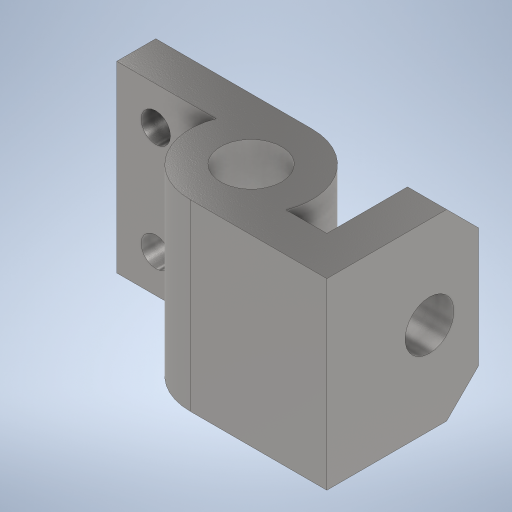
# Autodesk Inventor part: practice4
Saved by Autodesk Inventor 2024 (Build 280153000, 153)
## iProperties
Created: 2024-02-15
Part Number: practice4
Material: Stahl, galvanisiert
Document SubType Name: Modeling
Designer: ffogue
Density: 7.85 g/cm^3
Appearance: Galvanisiert
Author: ffogue
Autodesk Inventor part; units mm, degrees
ref_plane "YZ Plane" through (0, 0, 0) normal (1, 0, 0) x (0, 1, 0)
ref_plane "XZ Plane" through (0, 0, 0) normal (0, 1, 0) x (-1, 0, 0)
ref_plane "XY Plane" through (0, 0, 0) normal (0, 0, 1) x (1, 0, 0)
sketch "Skizze1" plane through (0, 0, 0) normal (0, 0, 1) x (1, 0, 0)
  line L0 (40, 37) -> (56, 37)
  line L1 (56, 37) -> (56, -25)
  line L2 (40, -9) -> (40, 37)
  line L3 (56, -25) -> (0, -25)
  line L4 (40, -9) -> (23.3238, -9)
  line L5 (0, 25) -> (-64, 25)
  line L6 (-64, 25) -> (-64, 9)
  line L7 (-64, 9) -> (-23.3238, 9)
  arc A0 (23.3238, -9) -> (0, 25) centre (0, 0) ccw
  arc A1 (-23.3238, 9) -> (0, -25) centre (0, 0) ccw
  dimension "d0" = 16
  dimension "d1" = 25
  dimension "d2" = 62
  dimension "d3" = 56
  dimension "d4" = 16
  dimension "d5" = 120
  dimension "d6" = 16
  dimension "d7" = 25
  constraints: 16 end point, 4 horizontal, 4 point on circle, 3 perpendicular, 2 centre point, 2 tangent, 1 coincident, 1 parallel
  measures "d0" distance between parallel lines of L3 L4
  measures "d1" distance from line of L3 A0.centre
  measures "d2" distance between parallel lines of L0 L3
  measures "d3" distance from line of L1 A0.centre
  measures "d4" distance between parallel lines of L1 L2
  measures "d5" distance between parallel lines of L1 L6
  measures "d6" distance between parallel lines of L7 L5
  measures "d7" radius of A0
extrude "Extrusion1" add sketch "Skizze1" along normal blind 75
sketch "Skizze2" plane through (0, 0, 75) normal (0, 0, 1) x (1, 0, 0)
  circle A0 centre (0, 0) radius 12.5
  dimension "d10" = 25
  constraints: 1 centre point, 1 coincident
  measures "d10" diameter of A0
extrude "Extrusion2" cut sketch "Skizze2" against normal up to surface (75 mm away)
chamfer "Fasen1" distance 13 angle 45 2 edges at (48, 37, 75) (48, 37, 0)
sketch "Skizze3" plane through (56, -25, 75) normal (1, 0, 0) x (0, 0, -1)
  line L0 (62, 62) -> (13, 62) projected
  point P0 (75, 25)
  point P1 (37.5, 42)
  point P2 (37.5, 62)
  dimension "d23" = 20
  constraints: 1 midpoint, 1 vertical alignment
  measures "d23" distance from line of point (37.5, 42) L0
hole "Bohrung1" at (56, 17, 37.5) direction (-1, 0, 0) diameter 20 depth 16
sketch "Skizze4" plane through (-64, 25, 0) normal (0, 1, 0) x (1, 0, 0)
  line L0 (0, 0) -> (0, -75) projected
  line L1 (0, -37.5) -> (64, -37.5) construction
  line L2 (64, 0) -> (64, -75) projected
  point P0 (16, -59.5)
  point P1 (16, -15.5)
  dimension "d31" = 44
  dimension "d32" = 16
  constraints: 2 end point, 2 midpoint, 1 symmetric about line
  measures "d31" distance of point (16, -15.5) point (16, -59.5)
  measures "d32" distance from line of L0 point (16, -59.5)
hole "Bohrung2" at (-48, 25, 59.5) at (-48, 25, 15.5) direction (0, -1, 0) diameter 12 end through all
equation "\"d0\" = d4"
equation "\"d6\" = d0"
